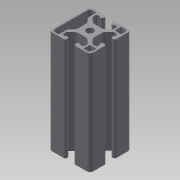
# Autodesk Inventor part: 40-4003
Saved by Autodesk Inventor 2013 (Build 170138000, 138)
## iProperties
Created: 2014-04-23
Part Number: 40-4003
Material: Generic
Document SubType Name: Modeling
Designer: Ross Bowman
Density: 1 g/cm^3
Engineer: Ross Bowman
Catalog Web Link: 8020.net
Vendor: 80/20 Inc.
Company: 80/20 Inc.
Author: Ross Bowman
Keywords: 80/20 , 8020 , T-Slot , Extrusion
Material: 6105-T5 Aluminum
Autodesk Inventor part; units mm, degrees
ref_plane "YZ Plane" through (0, 0, 0) normal (1, 0, 0) x (0, 1, 0)
ref_plane "XZ Plane" through (0, 0, 0) normal (0, 1, 0) x (-1, 0, 0)
ref_plane "XY Plane" through (0, 0, 0) normal (0, 0, 1) x (1, 0, 0)
sketch "Sketch1" plane through (0, 0, 0) normal (0, 0, 1) x (1, 0, 0)
  arc A0 (11.9044, -17.715) -> (12.5394, -18.35) centre (12.5394, -17.715) ccw
  line L0 (11.9044, -13.3034) -> (11.9044, -17.715)
  arc A1 (13.1744, -12.0334) -> (11.9044, -13.3034) centre (13.1744, -13.3034) ccw
  line L1 (17.715, -12.0334) -> (13.1744, -12.0334)
  arc A2 (18.35, -12.6684) -> (17.715, -12.0334) centre (17.715, -12.6684) ccw
  line L2 (18.35, -15.556) -> (18.35, -12.6684)
  arc A3 (15.556, -18.35) -> (18.35, -15.556) centre (15.556, -15.556) ccw
  line L3 (12.5394, -18.35) -> (15.556, -18.35)
  arc A4 (-12.566, -18.35) -> (-11.9311, -17.7218) centre (-12.566, -17.715) ccw
  line L4 (-15.556, -18.35) -> (-12.566, -18.35)
  arc A5 (-18.35, -15.5575) -> (-15.556, -18.35) centre (-15.556, -15.556) ccw
  line L5 (-18.35, 15.5575) -> (-18.35, -15.5575)
  arc A6 (-15.556, 18.35) -> (-18.35, 15.5575) centre (-15.556, 15.556) ccw
  line L6 (-12.566, 18.35) -> (-15.556, 18.35)
  arc A7 (-11.9311, 17.7218) -> (-12.566, 18.35) centre (-12.566, 17.715) ccw
  line L7 (-11.9311, 10.9555) -> (-11.9311, 17.7218)
  arc A8 (-11.9311, 10.9555) -> (-11.0096, 8.5897) centre (-8.7586, 10.8288) ccw
  line L8 (-9.0762, 6.6563) -> (-11.0096, 8.5897)
  arc A9 (-7.685, 3.2977) -> (-9.0762, 6.6563) centre (-12.4348, 3.2977) ccw
  line L9 (-7.685, -3.4647) -> (-7.685, 3.2977)
  arc A10 (-9.112, -6.8083) -> (-7.685, -3.4647) centre (-12.4345, -3.414) ccw
  line L10 (-11.066, -8.7209) -> (-9.112, -6.8083)
  arc A11 (-11.066, -8.7209) -> (-11.9311, -10.9555) centre (-8.7566, -10.8997) ccw
  line L11 (-11.9311, -17.7218) -> (-11.9311, -10.9555)
  circle A12 centre (0, 0) radius 3.4
  arc A13 (11.9044, 13.3034) -> (13.1744, 12.0334) centre (13.1744, 13.3034) ccw
  line L12 (11.9044, 17.715) -> (11.9044, 13.3034)
  arc A14 (12.5394, 18.35) -> (11.9044, 17.715) centre (12.5394, 17.715) ccw
  line L13 (15.556, 18.35) -> (12.5394, 18.35)
  arc A15 (18.35, 15.556) -> (15.556, 18.35) centre (15.556, 15.556) ccw
  line L14 (18.35, 12.6684) -> (18.35, 15.556)
  arc A16 (17.715, 12.0334) -> (18.35, 12.6684) centre (17.715, 12.6684) ccw
  line L15 (13.1744, 12.0334) -> (17.715, 12.0334)
  arc A17 (3.5467, 7.685) -> (6.8256, 9.1591) centre (3.3834, 12.432) ccw
  line L16 (3.5467, 7.685) -> (-3.2157, 7.685)
  arc A18 (-6.7073, 9.2147) -> (-3.2157, 7.685) centre (-3.2157, 12.4348) ccw
  line L17 (-6.7073, 9.2147) -> (-9.9941, 12.5015)
  arc A19 (-10.2545, 13.1301) -> (-9.9941, 12.5015) centre (-9.3655, 13.1301) ccw
  line L18 (-10.2545, 13.1301) -> (-10.2545, 15.4285)
  arc A20 (-8.9845, 16.6985) -> (-10.2545, 15.4285) centre (-8.9845, 15.4285) ccw
  line L19 (-8.9845, 16.6985) -> (-6.7752, 16.6985)
  line L20 (-6.7752, 16.6985) -> (-6.7752, 15.936)
  line L21 (-6.7752, 15.936) -> (-5.6348, 15.936)
  arc A21 (-5.6348, 15.936) -> (-4.06, 17.5108) centre (-5.6348, 17.5108) ccw
  line L22 (-4.06, 17.5108) -> (-4.06, 18.4252)
  arc A22 (-4.06, 18.4252) -> (-5.6348, 20) centre (-5.6348, 18.4252) ccw
  line L23 (-5.6348, 20) -> (-16.825, 20)
  arc A23 (-16.825, 20) -> (-20, 16.825) centre (-16.825, 16.825) ccw
  line L24 (-20, 16.825) -> (-20, -16.825)
  arc A24 (-20, -16.825) -> (-16.825, -20) centre (-16.825, -16.825) ccw
  line L25 (-16.825, -20) -> (-5.6348, -20)
  arc A25 (-5.6348, -20) -> (-4.06, -18.4252) centre (-5.6348, -18.4252) ccw
  line L26 (-4.06, -18.4252) -> (-4.06, -17.5108)
  arc A26 (-4.06, -17.5108) -> (-5.6348, -15.936) centre (-5.6348, -17.5108) ccw
  line L27 (-5.6348, -15.936) -> (-6.7752, -15.936)
  line L28 (-6.7752, -15.936) -> (-6.7752, -16.6985)
  line L29 (-6.7752, -16.6985) -> (-8.9845, -16.6985)
  arc A27 (-10.2545, -15.4285) -> (-8.9845, -16.6985) centre (-8.9845, -15.4285) ccw
  line L30 (-10.2545, -15.4285) -> (-10.2545, -13.1306)
  arc A28 (-9.9941, -12.5019) -> (-10.2545, -13.1306) centre (-9.3655, -13.1306) ccw
  line L31 (-9.9941, -12.5019) -> (-6.7073, -9.2151)
  arc A29 (-3.2152, -7.685) -> (-6.7073, -9.2151) centre (-3.2152, -12.4348) ccw
  line L32 (-3.2152, -7.685) -> (3.3848, -7.685)
  arc A30 (6.7926, -9.126) -> (3.3848, -7.685) centre (3.3848, -12.4348) ccw
  line L33 (6.7926, -9.126) -> (9.994, -12.3275)
  arc A31 (10.2544, -12.9561) -> (9.994, -12.3275) centre (9.3654, -12.9561) ccw
  line L34 (10.2544, -12.9561) -> (10.2544, -15.4395)
  arc A32 (8.9845, -16.6985) -> (10.2544, -15.4395) centre (8.9845, -15.4285) ccw
  line L35 (8.9845, -16.6985) -> (6.7752, -16.6985)
  line L36 (6.7752, -16.6985) -> (6.7752, -15.936)
  line L37 (6.7752, -15.936) -> (5.6348, -15.936)
  arc A33 (5.6348, -15.936) -> (4.06, -17.5108) centre (5.6348, -17.5108) ccw
  line L38 (4.06, -17.5108) -> (4.06, -18.4252)
  arc A34 (4.06, -18.4252) -> (5.6348, -20) centre (5.6348, -18.4252) ccw
  line L39 (5.6348, -20) -> (17.1517, -20)
  arc A35 (17.1517, -20) -> (20, -16.825) centre (16.825, -16.8418) ccw
  line L40 (20, -16.825) -> (20, -5.5728)
  arc A36 (20, -5.5728) -> (18.4264, -4.06) centre (18.4264, -5.6348) ccw
  line L41 (18.4264, -4.06) -> (17.5148, -4.06)
  arc A37 (17.5148, -4.06) -> (15.94, -5.6348) centre (17.5148, -5.6348) ccw
  line L42 (15.94, -5.6348) -> (15.94, -6.7752)
  line L43 (15.94, -6.7752) -> (16.7025, -6.7752)
  line L44 (16.7025, -6.7752) -> (16.7025, -8.9845)
  arc A38 (15.383, -10.3834) -> (16.7025, -8.9845) centre (15.4392, -9.1146) ccw
  line L45 (15.383, -10.3834) -> (13.0851, -10.3834)
  arc A39 (12.4565, -10.123) -> (13.0851, -10.3834) centre (13.0851, -9.4944) ccw
  line L46 (12.4565, -10.123) -> (9.1697, -6.8362)
  arc A40 (7.685, -3.5711) -> (9.1697, -6.8362) centre (12.4311, -3.3831) ccw
  line L47 (7.685, -3.5711) -> (7.685, 3.1913)
  arc A41 (8.9798, 6.6463) -> (7.685, 3.1913) centre (12.4309, 3.3829) ccw
  line L48 (8.9798, 6.6463) -> (12.2666, 9.9331)
  arc A42 (13.0398, 10.3834) -> (12.2666, 9.9331) centre (13.0398, 9.4944) ccw
  line L49 (13.0398, 10.3834) -> (15.3781, 10.3834)
  arc A43 (16.6462, 9.1821) -> (15.3781, 10.3834) centre (15.3781, 9.1134) ccw
  line L50 (16.6462, 9.1821) -> (16.6462, 6.9728)
  line L51 (16.6462, 6.9728) -> (15.94, 6.9728)
  line L52 (15.94, 6.9728) -> (15.94, 5.8324)
  arc A44 (15.94, 5.8324) -> (17.5024, 4.06) centre (17.5024, 5.6348) ccw
  line L53 (17.5024, 4.06) -> (18.4252, 4.06)
  arc A45 (18.4252, 4.06) -> (20, 5.6348) centre (18.4252, 5.6348) ccw
  line L54 (20, 5.6348) -> (20, 16.8242)
  arc A46 (20, 16.8242) -> (16.825, 20) centre (16.825, 16.825) ccw
  line L55 (16.825, 20) -> (5.6348, 20)
  arc A47 (5.6348, 20) -> (4.06, 18.4252) centre (5.6348, 18.4252) ccw
  line L56 (4.06, 18.4252) -> (4.06, 17.5108)
  arc A48 (4.06, 17.5108) -> (5.6348, 15.936) centre (5.6348, 17.5108) ccw
  line L57 (5.6348, 15.936) -> (6.7752, 15.936)
  line L58 (6.7752, 15.936) -> (6.7752, 16.6985)
  line L59 (6.7752, 16.6985) -> (8.9845, 16.6985)
  arc A49 (10.3155, 15.4299) -> (8.9845, 16.6985) centre (9.0455, 15.4299) ccw
  line L60 (10.3155, 15.4299) -> (10.3155, 13.1309)
  arc A50 (10.1069, 12.4403) -> (10.3155, 13.1309) centre (9.4334, 13.0206) ccw
  line L61 (10.1069, 12.4403) -> (6.8256, 9.1591)
  constraints: 124 end point, 100 point on circle, 51 centre point
extrude "Extrusion1" add sketch "Sketch1" against normal blind 100
body "Solid1"
